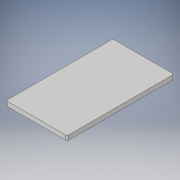
# Autodesk Inventor part: Spielstraßenschild_Teil_Oben
Saved by Autodesk Inventor 2019.5 (Build 235369000, 369)
## iProperties
Created: 2021-10-06
Part Number: Spielstraßenschild_Teil_Oben
Material: Generisch
Document SubType Name: Modeling
Designer: mritt
Density: 1 g/cm^3
Appearance: Vorgabe
Author: mritt
Autodesk Inventor part; units mm, degrees
ref_plane "YZ Plane" through (0, 0, 0) normal (1, 0, 0) x (0, 1, 0)
ref_plane "XZ Plane" through (0, 0, 0) normal (0, 1, 0) x (-1, 0, 0)
ref_plane "XY Plane" through (0, 0, 0) normal (0, 0, 1) x (1, 0, 0)
sketch "Skizze1" plane through (0, 0, 0) normal (0, 1, 0) x (-1, 0, 0)
  line L0 (37.9316, -16.2735) -> (-2.0684, -16.2735)
  line L1 (-2.0684, -16.2735) -> (-2.0684, -86.2735)
  line L2 (-2.0684, -86.2735) -> (37.9316, -86.2735)
  line L3 (37.9316, -86.2735) -> (37.9316, -16.2735)
  point P0 (0, 0)
  dimension "d0" = 70
  dimension "d1" = 40
  constraints: 8 end point, 2 parallel, 1 horizontal, 1 perpendicular
  measures "d0" distance of L2.end L0.start
  measures "d1" distance of L1.end L2.end
extrude "Extrusion1" add sketch "Skizze1" along normal blind 3
fillet "Rundung1" radius 1 4 edges at (-37.9316, 1.5, -16.2735) (-37.9316, 1.5, -86.2735) (2.0684, 1.5, -86.2735) (2.0684, 1.5, -16.2735)
